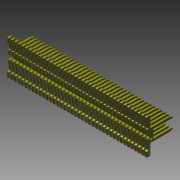
# Autodesk Inventor part: ST4-40-1.00-L-D_pin
Saved by Autodesk Inventor 2016 (Build 200138000, 138)
## iProperties
Category: PARTsolutions
Company: SAMTEC
Created: 2016-06-07
Part Number: ST4-40-1.00-L-D_pin
Catalog Web Link: www.cadenas.de
Description: ST4 Series Pin-ST4 Series - (0,40 mm) .0158" Razor Beam™ LP Ultra Fine Pitch Header & Socket
Vendor: SAMTEC
Document SubType Name: Modeling
Designer: psAdmin
Manufacturer: SAMTEC
Mass: 0.0199119 g
Surface Area: 3.75275 cm^2
Volume: 0.0199119 cm^3
Density: 1 g/cm^3
Material: Generic
Appearance: PSOLRGB-255-255-0
PSOL_IDENT_0: {$CADENAS_DATA\23d-libs\samtec\modelling\st4\parts\st4_pin.prj},199 {VTYP=3D},{NB=ST4-40-1.00-L-D_pi
PSOL_IDENT_1: n},{LINA=ST4-40-1.00-L-D_pin},{NN=ST4 Series Pin},{DATE=15.03.2016 09:56:18},{GEOMDATE=15.03.2016 09
PSOL_IDENT_2: :55:00},{VERSION=},{LINEID=10},{LINESUBID=-1},{WBVAR=POS,LS,LOPT}  {NB=ST4-40-1.00-L-D_pin},{LINA=ST
PSOL_IDENT_3: 4-40-1.00-L-D_pin},{KT=DUMMY},{SERIES=ST4},{PN=ST4-40-1.00-L-D},{POS=40},{POSATOF=40},{LS=1.00},{PLO
PSOL_IDENT_4: PT=-L: 10micro\" Selective Gold in Contact Area, Matte Tin on Tail},{ROW=-D: Double},{LOPT=},{LOPTAL
PSOL_IDENT_5: G= '','Not Selected','L','-L: Latching' },{LOPTPN=},{A=16.25},{B=15.6},{C=17.4},{F=22.46},{H=19.9},{
PSOL_IDENT_6: J=19.5},{D=3.55},{L=3.58},{DP=0.68000},{TP=2.76000},{PP=0.32000}
NN: ST4 Series Pin
NT: ST4 Series - (0,40 mm) .0158" Razor Beam™ LP Ultra Fine Pitch Header & Socket
NB: ST4-40-1.00-L-D_pin
NBSYN: $PN._pin
LINA: ST4-40-1.00-L-D_pin
SERIES: ST4
POS: 40
LS: 1.00
PLOPT: -L: 10micro" Selective Gold in Contact Area, Matte Tin on Tail
ROW: -D: Double
LOPT: Not Selected
SUPPLIER: SAMTEC
ARTICLENO: ST4-40-1.00-L-D_pin
BOMINFO: ST4-40-1.00-L-D_pin
CREATOR: CADENAS GmbH
Title: ST4-40-1.00-L-D_pin
Author: Cadenas PARTsolutions
Comments: ST4 Series - (0,40 mm) .0158" Razor Beam™ LP Ultra Fine Pitch Header & Socket
Autodesk Inventor part; units mm, degrees
sketch "Sketch_1" plane through (0, 0, 0) normal (0, 0, 1) x (1, 0, 0)
  line L0 (-7.9, 3.08) -> (-7.9, 0)
  line L1 (-7.9, 0) -> (-7.7, 0)
  line L2 (-7.7, 0) -> (-7.7, 0.72)
  line L3 (-7.7, 0.72) -> (-7.5, 0.72)
  line L4 (-7.5, 0.72) -> (-7.5, 0)
  line L5 (-7.5, 0) -> (-7.3, 0)
  line L6 (-7.3, 0) -> (-7.3, 0.72)
  line L7 (-7.3, 0.72) -> (-7.1, 0.72)
  line L8 (-7.1, 0.72) -> (-7.1, 0)
  line L9 (-7.1, 0) -> (-6.9, 0)
  line L10 (-6.9, 0) -> (-6.9, 0.72)
  line L11 (-6.9, 0.72) -> (-6.7, 0.72)
  line L12 (-6.7, 0.72) -> (-6.7, 0)
  line L13 (-6.7, 0) -> (-6.5, 0)
  line L14 (-6.5, 0) -> (-6.5, 0.72)
  line L15 (-6.5, 0.72) -> (-6.3, 0.72)
  line L16 (-6.3, 0.72) -> (-6.3, 0)
  line L17 (-6.3, 0) -> (-6.1, 0)
  line L18 (-6.1, 0) -> (-6.1, 0.72)
  line L19 (-6.1, 0.72) -> (-5.9, 0.72)
  line L20 (-5.9, 0.72) -> (-5.9, 0)
  line L21 (-5.9, 0) -> (-5.7, 0)
  line L22 (-5.7, 0) -> (-5.7, 0.72)
  line L23 (-5.7, 0.72) -> (-5.5, 0.72)
  line L24 (-5.5, 0.72) -> (-5.5, 0)
  line L25 (-5.5, 0) -> (-5.3, 0)
  line L26 (-5.3, 0) -> (-5.3, 0.72)
  line L27 (-5.3, 0.72) -> (-5.1, 0.72)
  line L28 (-5.1, 0.72) -> (-5.1, 0)
  line L29 (-5.1, 0) -> (-4.9, 0)
  line L30 (-4.9, 0) -> (-4.9, 0.72)
  line L31 (-4.9, 0.72) -> (-4.7, 0.72)
  line L32 (-4.7, 0.72) -> (-4.7, 0)
  line L33 (-4.7, 0) -> (-4.5, 0)
  line L34 (-4.5, 0) -> (-4.5, 0.72)
  line L35 (-4.5, 0.72) -> (-4.3, 0.72)
  line L36 (-4.3, 0.72) -> (-4.3, 0)
  line L37 (-4.3, 0) -> (-4.1, 0)
  line L38 (-4.1, 0) -> (-4.1, 0.72)
  line L39 (-4.1, 0.72) -> (-3.9, 0.72)
  line L40 (-3.9, 0.72) -> (-3.9, 0)
  line L41 (-3.9, 0) -> (-3.7, 0)
  line L42 (-3.7, 0) -> (-3.7, 0.72)
  line L43 (-3.7, 0.72) -> (-3.5, 0.72)
  line L44 (-3.5, 0.72) -> (-3.5, 0)
  line L45 (-3.5, 0) -> (-3.3, 0)
  line L46 (-3.3, 0) -> (-3.3, 0.72)
  line L47 (-3.3, 0.72) -> (-3.1, 0.72)
  line L48 (-3.1, 0.72) -> (-3.1, 0)
  line L49 (-3.1, 0) -> (-2.9, 0)
  line L50 (-2.9, 0) -> (-2.9, 0.72)
  line L51 (-2.9, 0.72) -> (-2.7, 0.72)
  line L52 (-2.7, 0.72) -> (-2.7, 0)
  line L53 (-2.7, 0) -> (-2.5, 0)
  line L54 (-2.5, 0) -> (-2.5, 0.72)
  line L55 (-2.5, 0.72) -> (-2.3, 0.72)
  line L56 (-2.3, 0.72) -> (-2.3, 0)
  line L57 (-2.3, 0) -> (-2.1, 0)
  line L58 (-2.1, 0) -> (-2.1, 0.72)
  line L59 (-2.1, 0.72) -> (-1.9, 0.72)
  line L60 (-1.9, 0.72) -> (-1.9, 0)
  line L61 (-1.9, 0) -> (-1.7, 0)
  line L62 (-1.7, 0) -> (-1.7, 0.72)
  line L63 (-1.7, 0.72) -> (-1.5, 0.72)
  line L64 (-1.5, 0.72) -> (-1.5, 0)
  line L65 (-1.5, 0) -> (-1.3, 0)
  line L66 (-1.3, 0) -> (-1.3, 0.72)
  line L67 (-1.3, 0.72) -> (-1.1, 0.72)
  line L68 (-1.1, 0.72) -> (-1.1, 0)
  line L69 (-1.1, 0) -> (-0.9, 0)
  line L70 (-0.9, 0) -> (-0.9, 0.72)
  line L71 (-0.9, 0.72) -> (-0.7, 0.72)
  line L72 (-0.7, 0.72) -> (-0.7, 0)
  line L73 (-0.7, 0) -> (-0.5, 0)
  line L74 (-0.5, 0) -> (-0.5, 0.72)
  line L75 (-0.5, 0.72) -> (-0.3, 0.72)
  line L76 (-0.3, 0.72) -> (-0.3, 0)
  line L77 (-0.3, 0) -> (-0.1, 0)
  line L78 (-0.1, 0) -> (-0.1, 0.72)
  line L79 (-0.1, 0.72) -> (0.1, 0.72)
  line L80 (0.1, 0.72) -> (0.1, 0)
  line L81 (0.1, 0) -> (0.3, 0)
  line L82 (0.3, 0) -> (0.3, 0.72)
  line L83 (0.3, 0.72) -> (0.5, 0.72)
  line L84 (0.5, 0.72) -> (0.5, 0)
  line L85 (0.5, 0) -> (0.7, 0)
  line L86 (0.7, 0) -> (0.7, 0.72)
  line L87 (0.7, 0.72) -> (0.9, 0.72)
  line L88 (0.9, 0.72) -> (0.9, 0)
  line L89 (0.9, 0) -> (1.1, 0)
  line L90 (1.1, 0) -> (1.1, 0.72)
  line L91 (1.1, 0.72) -> (1.3, 0.72)
  line L92 (1.3, 0.72) -> (1.3, 0)
  line L93 (1.3, 0) -> (1.5, 0)
  line L94 (1.5, 0) -> (1.5, 0.72)
  line L95 (1.5, 0.72) -> (1.7, 0.72)
  line L96 (1.7, 0.72) -> (1.7, 0)
  line L97 (1.7, 0) -> (1.9, 0)
  line L98 (1.9, 0) -> (1.9, 0.72)
  line L99 (1.9, 0.72) -> (2.1, 0.72)
  line L100 (2.1, 0.72) -> (2.1, 0)
  line L101 (2.1, 0) -> (2.3, 0)
  line L102 (2.3, 0) -> (2.3, 0.72)
  line L103 (2.3, 0.72) -> (2.5, 0.72)
  line L104 (2.5, 0.72) -> (2.5, 0)
  line L105 (2.5, 0) -> (2.7, 0)
  line L106 (2.7, 0) -> (2.7, 0.72)
  line L107 (2.7, 0.72) -> (2.9, 0.72)
  line L108 (2.9, 0.72) -> (2.9, 0)
  line L109 (2.9, 0) -> (3.1, 0)
  line L110 (3.1, 0) -> (3.1, 0.72)
  line L111 (3.1, 0.72) -> (3.3, 0.72)
  line L112 (3.3, 0.72) -> (3.3, 0)
  line L113 (3.3, 0) -> (3.5, 0)
  line L114 (3.5, 0) -> (3.5, 0.72)
  line L115 (3.5, 0.72) -> (3.7, 0.72)
  line L116 (3.7, 0.72) -> (3.7, 0)
  line L117 (3.7, 0) -> (3.9, 0)
  line L118 (3.9, 0) -> (3.9, 0.72)
  line L119 (3.9, 0.72) -> (4.1, 0.72)
  line L120 (4.1, 0.72) -> (4.1, 0)
  line L121 (4.1, 0) -> (4.3, 0)
  line L122 (4.3, 0) -> (4.3, 0.72)
  line L123 (4.3, 0.72) -> (4.5, 0.72)
  line L124 (4.5, 0.72) -> (4.5, 0)
  line L125 (4.5, 0) -> (4.7, 0)
  line L126 (4.7, 0) -> (4.7, 0.72)
  line L127 (4.7, 0.72) -> (4.9, 0.72)
  line L128 (4.9, 0.72) -> (4.9, 0)
  line L129 (4.9, 0) -> (5.1, 0)
  line L130 (5.1, 0) -> (5.1, 0.72)
  line L131 (5.1, 0.72) -> (5.3, 0.72)
  line L132 (5.3, 0.72) -> (5.3, 0)
  line L133 (5.3, 0) -> (5.5, 0)
  line L134 (5.5, 0) -> (5.5, 0.72)
  line L135 (5.5, 0.72) -> (5.7, 0.72)
  line L136 (5.7, 0.72) -> (5.7, 0)
  line L137 (5.7, 0) -> (5.9, 0)
  line L138 (5.9, 0) -> (5.9, 0.72)
  line L139 (5.9, 0.72) -> (6.1, 0.72)
  line L140 (6.1, 0.72) -> (6.1, 0)
  line L141 (6.1, 0) -> (6.3, 0)
  line L142 (6.3, 0) -> (6.3, 0.72)
  line L143 (6.3, 0.72) -> (6.5, 0.72)
  line L144 (6.5, 0.72) -> (6.5, 0)
  line L145 (6.5, 0) -> (6.7, 0)
  line L146 (6.7, 0) -> (6.7, 0.72)
  line L147 (6.7, 0.72) -> (6.9, 0.72)
  line L148 (6.9, 0.72) -> (6.9, 0)
  line L149 (6.9, 0) -> (7.1, 0)
  line L150 (7.1, 0) -> (7.1, 0.72)
  line L151 (7.1, 0.72) -> (7.3, 0.72)
  line L152 (7.3, 0.72) -> (7.3, 0)
  line L153 (7.3, 0) -> (7.5, 0)
  line L154 (7.5, 0) -> (7.5, 0.72)
  line L155 (7.5, 0.72) -> (7.7, 0.72)
  line L156 (7.7, 0.72) -> (7.7, 0)
  line L157 (7.7, 0) -> (7.9, 0)
  line L158 (7.9, 0) -> (7.9, 3.08)
  line L159 (7.9, 3.08) -> (7.7, 3.08)
  line L160 (7.7, 3.08) -> (7.7, 0.77)
  line L161 (7.7, 0.77) -> (7.5, 0.77)
  line L162 (7.5, 0.77) -> (7.5, 3.08)
  line L163 (7.5, 3.08) -> (7.3, 3.08)
  line L164 (7.3, 3.08) -> (7.3, 0.77)
  line L165 (7.3, 0.77) -> (7.1, 0.77)
  line L166 (7.1, 0.77) -> (7.1, 3.08)
  line L167 (7.1, 3.08) -> (6.9, 3.08)
  line L168 (6.9, 3.08) -> (6.9, 0.77)
  line L169 (6.9, 0.77) -> (6.7, 0.77)
  line L170 (6.7, 0.77) -> (6.7, 3.08)
  line L171 (6.7, 3.08) -> (6.5, 3.08)
  line L172 (6.5, 3.08) -> (6.5, 0.77)
  line L173 (6.5, 0.77) -> (6.3, 0.77)
  line L174 (6.3, 0.77) -> (6.3, 3.08)
  line L175 (6.3, 3.08) -> (6.1, 3.08)
  line L176 (6.1, 3.08) -> (6.1, 0.77)
  line L177 (6.1, 0.77) -> (5.9, 0.77)
  line L178 (5.9, 0.77) -> (5.9, 3.08)
  line L179 (5.9, 3.08) -> (5.7, 3.08)
  line L180 (5.7, 3.08) -> (5.7, 0.77)
  line L181 (5.7, 0.77) -> (5.5, 0.77)
  line L182 (5.5, 0.77) -> (5.5, 3.08)
  line L183 (5.5, 3.08) -> (5.3, 3.08)
  line L184 (5.3, 3.08) -> (5.3, 0.77)
  line L185 (5.3, 0.77) -> (5.1, 0.77)
  line L186 (5.1, 0.77) -> (5.1, 3.08)
  line L187 (5.1, 3.08) -> (4.9, 3.08)
  line L188 (4.9, 3.08) -> (4.9, 0.77)
  line L189 (4.9, 0.77) -> (4.7, 0.77)
  line L190 (4.7, 0.77) -> (4.7, 3.08)
  line L191 (4.7, 3.08) -> (4.5, 3.08)
  line L192 (4.5, 3.08) -> (4.5, 0.77)
  line L193 (4.5, 0.77) -> (4.3, 0.77)
  line L194 (4.3, 0.77) -> (4.3, 3.08)
  line L195 (4.3, 3.08) -> (4.1, 3.08)
  line L196 (4.1, 3.08) -> (4.1, 0.77)
  line L197 (4.1, 0.77) -> (3.9, 0.77)
  line L198 (3.9, 0.77) -> (3.9, 3.08)
  line L199 (3.9, 3.08) -> (3.7, 3.08)
  line L200 (3.7, 3.08) -> (3.7, 0.77)
  line L201 (3.7, 0.77) -> (3.5, 0.77)
  line L202 (3.5, 0.77) -> (3.5, 3.08)
  line L203 (3.5, 3.08) -> (3.3, 3.08)
  line L204 (3.3, 3.08) -> (3.3, 0.77)
  line L205 (3.3, 0.77) -> (3.1, 0.77)
  line L206 (3.1, 0.77) -> (3.1, 3.08)
  line L207 (3.1, 3.08) -> (2.9, 3.08)
  line L208 (2.9, 3.08) -> (2.9, 0.77)
  line L209 (2.9, 0.77) -> (2.7, 0.77)
  line L210 (2.7, 0.77) -> (2.7, 3.08)
  line L211 (2.7, 3.08) -> (2.5, 3.08)
  line L212 (2.5, 3.08) -> (2.5, 0.77)
  line L213 (2.5, 0.77) -> (2.3, 0.77)
  line L214 (2.3, 0.77) -> (2.3, 3.08)
  line L215 (2.3, 3.08) -> (2.1, 3.08)
  line L216 (2.1, 3.08) -> (2.1, 0.77)
  line L217 (2.1, 0.77) -> (1.9, 0.77)
  line L218 (1.9, 0.77) -> (1.9, 3.08)
  line L219 (1.9, 3.08) -> (1.7, 3.08)
  line L220 (1.7, 3.08) -> (1.7, 0.77)
  line L221 (1.7, 0.77) -> (1.5, 0.77)
  line L222 (1.5, 0.77) -> (1.5, 3.08)
  line L223 (1.5, 3.08) -> (1.3, 3.08)
  line L224 (1.3, 3.08) -> (1.3, 0.77)
  line L225 (1.3, 0.77) -> (1.1, 0.77)
  line L226 (1.1, 0.77) -> (1.1, 3.08)
  line L227 (1.1, 3.08) -> (0.9, 3.08)
  line L228 (0.9, 3.08) -> (0.9, 0.77)
  line L229 (0.9, 0.77) -> (0.7, 0.77)
  line L230 (0.7, 0.77) -> (0.7, 3.08)
  line L231 (0.7, 3.08) -> (0.5, 3.08)
  line L232 (0.5, 3.08) -> (0.5, 0.77)
  line L233 (0.5, 0.77) -> (0.3, 0.77)
  line L234 (0.3, 0.77) -> (0.3, 3.08)
  line L235 (0.3, 3.08) -> (0.1, 3.08)
  line L236 (0.1, 3.08) -> (0.1, 0.77)
  line L237 (0.1, 0.77) -> (-0.1, 0.77)
  line L238 (-0.1, 0.77) -> (-0.1, 3.08)
  line L239 (-0.1, 3.08) -> (-0.3, 3.08)
  line L240 (-0.3, 3.08) -> (-0.3, 0.77)
  line L241 (-0.3, 0.77) -> (-0.5, 0.77)
  line L242 (-0.5, 0.77) -> (-0.5, 3.08)
  line L243 (-0.5, 3.08) -> (-0.7, 3.08)
  line L244 (-0.7, 3.08) -> (-0.7, 0.77)
  line L245 (-0.7, 0.77) -> (-0.9, 0.77)
  line L246 (-0.9, 0.77) -> (-0.9, 3.08)
  line L247 (-0.9, 3.08) -> (-1.1, 3.08)
  line L248 (-1.1, 3.08) -> (-1.1, 0.77)
  line L249 (-1.1, 0.77) -> (-1.3, 0.77)
  line L250 (-1.3, 0.77) -> (-1.3, 3.08)
  line L251 (-1.3, 3.08) -> (-1.5, 3.08)
  line L252 (-1.5, 3.08) -> (-1.5, 0.77)
  line L253 (-1.5, 0.77) -> (-1.7, 0.77)
  line L254 (-1.7, 0.77) -> (-1.7, 3.08)
  line L255 (-1.7, 3.08) -> (-1.9, 3.08)
  line L256 (-1.9, 3.08) -> (-1.9, 0.77)
  line L257 (-1.9, 0.77) -> (-2.1, 0.77)
  line L258 (-2.1, 0.77) -> (-2.1, 3.08)
  line L259 (-2.1, 3.08) -> (-2.3, 3.08)
  line L260 (-2.3, 3.08) -> (-2.3, 0.77)
  line L261 (-2.3, 0.77) -> (-2.5, 0.77)
  line L262 (-2.5, 0.77) -> (-2.5, 3.08)
  line L263 (-2.5, 3.08) -> (-2.7, 3.08)
  line L264 (-2.7, 3.08) -> (-2.7, 0.77)
  line L265 (-2.7, 0.77) -> (-2.9, 0.77)
  line L266 (-2.9, 0.77) -> (-2.9, 3.08)
  line L267 (-2.9, 3.08) -> (-3.1, 3.08)
  line L268 (-3.1, 3.08) -> (-3.1, 0.77)
  line L269 (-3.1, 0.77) -> (-3.3, 0.77)
  line L270 (-3.3, 0.77) -> (-3.3, 3.08)
  line L271 (-3.3, 3.08) -> (-3.5, 3.08)
  line L272 (-3.5, 3.08) -> (-3.5, 0.77)
  line L273 (-3.5, 0.77) -> (-3.7, 0.77)
  line L274 (-3.7, 0.77) -> (-3.7, 3.08)
  line L275 (-3.7, 3.08) -> (-3.9, 3.08)
  line L276 (-3.9, 3.08) -> (-3.9, 0.77)
  line L277 (-3.9, 0.77) -> (-4.1, 0.77)
  line L278 (-4.1, 0.77) -> (-4.1, 3.08)
  line L279 (-4.1, 3.08) -> (-4.3, 3.08)
  line L280 (-4.3, 3.08) -> (-4.3, 0.77)
  line L281 (-4.3, 0.77) -> (-4.5, 0.77)
  line L282 (-4.5, 0.77) -> (-4.5, 3.08)
  line L283 (-4.5, 3.08) -> (-4.7, 3.08)
  line L284 (-4.7, 3.08) -> (-4.7, 0.77)
  line L285 (-4.7, 0.77) -> (-4.9, 0.77)
  line L286 (-4.9, 0.77) -> (-4.9, 3.08)
  line L287 (-4.9, 3.08) -> (-5.1, 3.08)
  line L288 (-5.1, 3.08) -> (-5.1, 0.77)
  line L289 (-5.1, 0.77) -> (-5.3, 0.77)
  line L290 (-5.3, 0.77) -> (-5.3, 3.08)
  line L291 (-5.3, 3.08) -> (-5.5, 3.08)
  line L292 (-5.5, 3.08) -> (-5.5, 0.77)
  line L293 (-5.5, 0.77) -> (-5.7, 0.77)
  line L294 (-5.7, 0.77) -> (-5.7, 3.08)
  line L295 (-5.7, 3.08) -> (-5.9, 3.08)
  line L296 (-5.9, 3.08) -> (-5.9, 0.77)
  line L297 (-5.9, 0.77) -> (-6.1, 0.77)
  line L298 (-6.1, 0.77) -> (-6.1, 3.08)
  line L299 (-6.1, 3.08) -> (-6.3, 3.08)
  line L300 (-6.3, 3.08) -> (-6.3, 0.77)
  line L301 (-6.3, 0.77) -> (-6.5, 0.77)
  line L302 (-6.5, 0.77) -> (-6.5, 3.08)
  line L303 (-6.5, 3.08) -> (-6.7, 3.08)
  line L304 (-6.7, 3.08) -> (-6.7, 0.77)
  line L305 (-6.7, 0.77) -> (-6.9, 0.77)
  line L306 (-6.9, 0.77) -> (-6.9, 3.08)
  line L307 (-6.9, 3.08) -> (-7.1, 3.08)
  line L308 (-7.1, 3.08) -> (-7.1, 0.77)
  line L309 (-7.1, 0.77) -> (-7.3, 0.77)
  line L310 (-7.3, 0.77) -> (-7.3, 3.08)
  line L311 (-7.3, 3.08) -> (-7.5, 3.08)
  line L312 (-7.5, 3.08) -> (-7.5, 0.77)
  line L313 (-7.5, 0.77) -> (-7.7, 0.77)
  line L314 (-7.7, 0.77) -> (-7.7, 3.08)
  line L315 (-7.7, 3.08) -> (-7.9, 3.08)
  constraints: 632 end point
extrude "Extrusion1" add sketch "Sketch_1" along normal mid plane 4.2
sketch "Sketch_2" plane through (0, 0, 0) normal (1, 0, 0) x (0, 1, 0)
  line L0 (-1, 3) -> (-1, -3)
  line L1 (-1, -3) -> (3.55, -3)
  line L2 (3.55, -3) -> (3.55, 3)
  line L3 (3.55, 3) -> (-1, 3)
  line L4 (0.345, 2) -> (0.08, 2)
  arc A0 (0.08, 2) -> (0, 1.92) centre (0.08, 1.92) ccw
  line L5 (0, 1.92) -> (0, 1.44)
  arc A1 (0, 1.44) -> (0.08, 1.36) centre (0.08, 1.44) ccw
  line L6 (0.08, 1.36) -> (0.1, 1.36)
  arc A2 (0.2, 1.26) -> (0.1, 1.36) centre (0.1, 1.26) ccw
  line L7 (0.2, 1.26) -> (0.2, 0.83)
  arc A3 (0.15, 0.7434) -> (0.2, 0.83) centre (0.1, 0.83) ccw
  arc A4 (0.1, 0.73) -> (0.15, 0.7434) centre (0.1, 0.83) ccw
  line L8 (0.1, 0.73) -> (0.1, 0.23)
  line L9 (0.1, 0.23) -> (0.425, 0.23)
  line L10 (0.425, 0.23) -> (0.425, 0.48)
  line L11 (0.425, 0.48) -> (0.72, 0.48)
  line L12 (0.72, 0.48) -> (0.72, -0.48)
  line L13 (0.72, -0.48) -> (0.425, -0.48)
  line L14 (0.425, -0.48) -> (0.425, -0.23)
  line L15 (0.425, -0.23) -> (0.1, -0.23)
  line L16 (0.1, -0.23) -> (0.1, -0.73)
  arc A5 (0.15, -0.7434) -> (0.1, -0.73) centre (0.1, -0.83) ccw
  arc A6 (0.2, -0.83) -> (0.15, -0.7434) centre (0.1, -0.83) ccw
  line L17 (0.2, -0.83) -> (0.2, -1.26)
  arc A7 (0.1, -1.36) -> (0.2, -1.26) centre (0.1, -1.26) ccw
  line L18 (0.1, -1.36) -> (0.08, -1.36)
  arc A8 (0.08, -1.36) -> (0, -1.44) centre (0.08, -1.44) ccw
  line L19 (0, -1.44) -> (0, -1.92)
  arc A9 (0, -1.92) -> (0.08, -2) centre (0.08, -1.92) ccw
  line L20 (0.08, -2) -> (0.345, -2)
  arc A10 (0.345, -2) -> (0.425, -1.92) centre (0.345, -1.92) ccw
  line L21 (0.425, -1.92) -> (0.425, -0.73)
  line L22 (0.425, -0.73) -> (2.4658, -0.73)
  arc A11 (2.4658, -0.73) -> (2.5953, -0.713) centre (2.4658, -0.23) ccw
  line L23 (2.5953, -0.713) -> (2.9144, -0.6274)
  arc A12 (2.9144, -0.6274) -> (2.895, -0.48) centre (2.895, -0.555) ccw
  line L24 (2.895, -0.48) -> (0.77, -0.48)
  line L25 (0.77, -0.48) -> (0.77, 0.48)
  line L26 (0.77, 0.48) -> (2.895, 0.48)
  arc A13 (2.895, 0.48) -> (2.9144, 0.6274) centre (2.895, 0.555) ccw
  line L27 (2.9144, 0.6274) -> (2.5953, 0.713)
  arc A14 (2.5953, 0.713) -> (2.4658, 0.73) centre (2.4658, 0.23) ccw
  line L28 (2.4658, 0.73) -> (0.425, 0.73)
  line L29 (0.425, 0.73) -> (0.425, 1.92)
  arc A15 (0.425, 1.92) -> (0.345, 2) centre (0.345, 1.92) ccw
  constraints: 60 end point, 32 point on circle, 16 centre point
extrude "Extrusion2" cut sketch "Sketch_2" along normal mid plane 80
ref_plane "pin_XY" through (0, 0, 0) normal (0, 1, 0) x (1, 0, 0)
ref_plane "pin_YZ" through (0, 0, 0) normal (1, 0, 0) x (0, 0, -1)
ref_plane "pin_ZX" through (0, 0, 0) normal (0, 0, -1) x (0, 1, 0)
body "Solid1"
